Autodesk Inventor part; units mm, degrees
(part 2 of 2)
  measures "d20" diameter of A228
  measures "d21" diameter of A229
  measures "d22" diameter of A225
extrude "押し出し4" cut sketch "スケッチ2" against normal blind 10 contours L58 A225 L57 A224 | A224 L57 A225 L59 | L56 A225 L58 A224 | A226 L58 | L58 A226 L57 | A224 L59 A225 L56 | A227 L57 L59 | L59 A227 | L57 A226 | A227 L57 | A229 L56 | L56 A229 L58 | A228 L59 L56 | L56 A228 | L58 A229 | A228 L59 picked at (150.9192, 107.918) picked at (150.9192, 102.0822) picked at (145.2179, 107.4954) picked at (145.4313, 102.0279)
fillet "フィレット4" radius 1 8 edges at (150, 83.5525, 2) (150, 126.4478, 2) (147, 83.5525, 2) (147, 126.4478, 2) (127.0524, 106.5001, 2) (169.9476, 106.5001, 2) (127.0524, 103.5001, 2) (169.9476, 103.5001, 2)
fillet "フィレット5" radius 4 8 edges at (140.6418, 106.5001, 2) (156.3581, 106.5001, 2) (140.6418, 103.5001, 2) (156.3581, 103.5001, 2) (147, 97.142, 2) (147, 112.8583, 2) (150, 97.142, 2) (150, 112.8583, 2)
equation "\"d8\" = d6"
equation "\"d9\" = d7"
